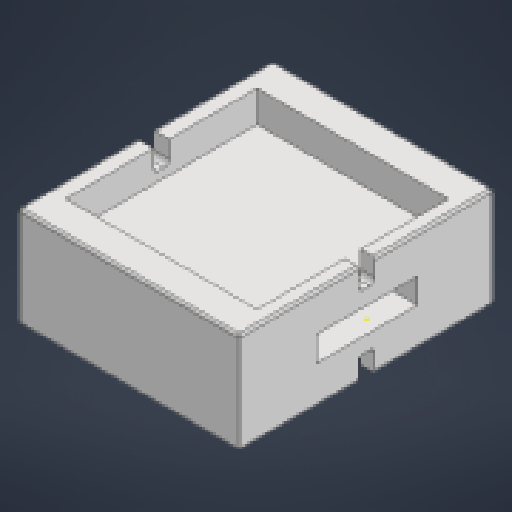
# Autodesk Inventor part: Base_Casing_A0645_v2
Saved by Autodesk Inventor 2026.2 (Build 302298000, 298)
## iProperties
Created: 2025-09-05
Part Number: Base_Casing_A0645_v2
Material: Generic
Document SubType Name: Modeling
Designer: usman
Density: 1 g/cm^3
Appearance: Default
Author: usman
Autodesk Inventor part; units mm, degrees
ref_plane "YZ Plane" through (0, 0, 0) normal (1, 0, 0) x (0, 1, 0)
ref_plane "XZ Plane" through (0, 0, 0) normal (0, 1, 0) x (-1, 0, 0)
ref_plane "XY Plane" through (0, 0, 0) normal (0, 0, 1) x (1, 0, 0)
sketch "Sketch1" plane through (0, 0, 0) normal (1, 0, 0) x (0, 1, 0)
  line L0 (-20, 51) -> (20, 51)
  line L1 (20, 51) -> (20, -51)
  line L2 (20, -51) -> (-20, -51)
  line L3 (-20, -51) -> (-20, 51)
  line L4 (-20, 51) -> (20, -51) construction
  line L5 (20, 51) -> (-20, -51) construction
  point P0 (0, 0)
  dimension "d0" = 40
  dimension "d30" = 102
  constraints: 12 end point, 2 midpoint, 2 parallel, 1 horizontal, 1 perpendicular
  measures "d0" distance of L1.end L2.end
  measures "d30" distance of L2.end L0.start
extrude "Extrusion1" add sketch "Sketch1" along normal blind 88.5
sketch "Sketch2" plane through (88.5, 0, 0) normal (1, 0, 0) x (0, 0, -1)
  line L0 (-20.32, -5) -> (20.32, -5)
  line L1 (20.32, -5) -> (20.32, 5)
  line L2 (20.32, 5) -> (-20.32, 5)
  line L3 (-20.32, 5) -> (-20.32, -5)
  line L4 (-20.32, -5) -> (20.32, 5) construction
  line L5 (20.32, -5) -> (-20.32, 5) construction
  point P0 (0, 0)
  dimension "d4" = 10
  dimension "d5" = 40.64
  constraints: 12 end point, 2 midpoint, 2 parallel, 1 horizontal, 1 perpendicular
  measures "d4" distance of L0.end L1.end
  measures "d5" distance of L1.end L2.end
extrude "Extrusion2" cut sketch "Sketch2" against normal through all
sketch "Sketch3" plane through (88.5, 0, 0) normal (1, 0, 0) x (0, 0, -1)
  point P0 (0, 0)
sketch "Sketch4" plane through (0, 20, 51) normal (0, 1, 0) x (1, 0, 0)
  line L0 (0, 102) -> (0, 0) projected
  line L1 (0, 102) -> (88.5, 102) projected
  line L2 (6.4418, 89.25) -> (82.9418, 89.25)
  line L3 (82.9418, 89.25) -> (82.9418, 12.75)
  line L4 (82.9418, 12.75) -> (6.4418, 12.75)
  line L5 (6.4418, 12.75) -> (6.4418, 89.25)
  line L6 (6.4418, 89.25) -> (82.9418, 12.75) construction
  line L7 (82.9418, 89.25) -> (6.4418, 12.75) construction
  line L8 (0, 0) -> (88.5, 0) projected
  point P0 (0, 51)
  point P1 (44.6918, 51)
  dimension "d24" = 102
  dimension "d31" = 76.5
  dimension "d32" = 76.5
  dimension "d34" = 51
  constraints: 12 end point, 2 parallel, 1 horizontal, 1 midpoint, 1 perpendicular
  measures "d24" distance of L0.start L0.end
  measures "d31" distance of L3.end L4.end
  measures "d32" distance of L2.end L3.end
  measures "d34" distance from line of L8 point (44.692, 51)
extrude "Extrusion3" cut sketch "Sketch4" against normal blind 12.5
mirror "Mirror1" about plane through (0, 0, 0) normal (0, 1, 0) of "Extrusion3"
sketch "Sketch5" plane through (0, 0, 0) normal (-1, 0, 0) x (0, 0, 1)
  line L0 (-51, 20) -> (51, 20) projected
  line L1 (-3.25, 11) -> (3.25, 11)
  line L2 (3.25, 11) -> (3.25, 20)
  line L3 (3.25, 20) -> (-3.25, 20)
  line L4 (-3.25, 20) -> (-3.25, 11)
  line L5 (-3.25, 11) -> (3.25, 20) construction
  line L6 (3.25, 11) -> (-3.25, 20) construction
  point P0 (0, 0)
  point P1 (0, 15.5)
  point P2 (-3.25, 20)
  dimension "d12" = 3.25
  dimension "d13" = 9
  constraints: 12 end point, 2 midpoint, 2 parallel, 1 horizontal, 1 perpendicular, 1 point on line
  measures "d12" distance from line of point (0, 15.5) L2
  measures "d13" distance of L1.end L2.end
extrude "Extrusion4" cut sketch "Sketch5" against normal through all
mirror "Mirror2" about plane through (0, 0, 0) normal (0, 1, 0) of "Extrusion4"
sketch "Sketch6" plane through (0, 0, 0) normal (-1, 0, 0) x (0, 0, 1)
  line L0 (-39.5306, -14.8221) -> (-39.5306, 14.9585) construction
  line L1 (-39.5306, 14.9585) -> (-30.121, 14.9585) construction
  line L2 (-30.121, 14.9585) -> (-30.121, -14.8221) construction
  line L3 (-30.121, -14.8221) -> (-39.5306, -14.8221) construction
  line L4 (-39.3809, -5.65) -> (-43.1909, -5.65)
  line L5 (-43.1909, -5.65) -> (-43.1909, -5.0532)
  spline S0 degree 2 poles (-43.1909, -5.0532) (-43.1909, -4.5318) (-43.125, -4.2899) knots 0 0 0 1 1 1
  spline S1 degree 2 poles (-43.125, -4.2899) (-43.0339, -3.9507) (-42.5407, -3.5455) (-42.2078, -3.5455) knots 0 0 0 1 2 2 2
  spline S2 degree 2 poles (-42.2078, -3.5455) (-41.9879, -3.5455) (-41.633, -3.7277) (-41.4791, -3.935) knots 0 0 0 1 2 2 2
  spline S3 degree 2 poles (-41.4791, -3.935) (-41.3158, -3.5863) (-40.8258, -3.266) (-40.4928, -3.266) knots 0 0 0 1 2 2 2
  spline S4 degree 2 poles (-40.4928, -3.266) (-40.1693, -3.266) (-39.6416, -3.5989) (-39.3809, -4.1203) (-39.3809, -4.582) knots 0 0 0 1 2 3 3 3
  line L6 (-39.3809, -4.582) -> (-39.3809, -5.65)
  line L7 (-41.0488, -4.9244) -> (-40.0719, -4.9244)
  line L8 (-40.0719, -4.9244) -> (-40.0719, -4.7422)
  spline S5 degree 2 poles (-40.0719, -4.7422) (-40.0719, -4.2931) (-40.3012, -3.979) (-40.518, -3.979) knots 0 0 0 1 2 2 2
  spline S6 degree 2 poles (-40.518, -3.979) (-40.7629, -3.979) (-41.0488, -4.3465) (-41.0488, -4.7736) knots 0 0 0 1 2 2 2
  line L9 (-41.0488, -4.7736) -> (-41.0488, -4.9244)
  line L10 (-42.4999, -4.9244) -> (-41.6958, -4.9244)
  line L11 (-41.6958, -4.9244) -> (-41.6958, -4.7673)
  spline S7 degree 2 poles (-41.6958, -4.7673) (-41.6958, -4.5035) (-41.9188, -4.2459) (-42.1104, -4.2459) knots 0 0 0 1 2 2 2
  spline S8 degree 2 poles (-42.1104, -4.2459) (-42.2895, -4.2459) (-42.4999, -4.4878) (-42.4999, -4.7391) knots 0 0 0 1 2 2 2
  line L12 (-42.4999, -4.7391) -> (-42.4999, -4.9244)
  line L13 (-42.1984, -0.571) -> (-42.1984, 0.1357)
  line L14 (-42.1984, 0.1357) -> (-39.3809, 0.1357)
  line L15 (-39.3809, 0.1357) -> (-39.3809, -0.571)
  line L16 (-39.3809, -0.571) -> (-39.6793, -0.571)
  spline S9 degree 2 poles (-39.6793, -0.571) (-39.4814, -0.7783) (-39.3087, -1.1929) (-39.3087, -1.4379) knots 0 0 0 1 2 2 2
  spline S10 degree 2 poles (-39.3087, -1.4379) (-39.3087, -1.9813) (-40.1567, -2.7791) (-40.7849, -2.7791) knots 0 0 0 1 2 2 2
  spline S11 degree 2 poles (-40.7849, -2.7791) (-41.4383, -2.7791) (-42.2706, -2.0096) (-42.2706, -1.4568) knots 0 0 0 1 2 2 2
  spline S12 degree 2 poles (-42.2706, -1.4568) (-42.2706, -1.2055) (-42.079, -0.7595) (-41.8874, -0.571) knots 0 0 0 1 2 2 2
  line L17 (-41.8874, -0.571) -> (-42.1984, -0.571)
  spline S13 degree 2 poles (-41.6173, -1.3154) (-41.6173, -1.6421) (-41.1556, -2.0755) (-40.7912, -2.0755) knots 0 0 0 1 2 2 2
  spline S14 degree 2 poles (-40.7912, -2.0755) (-40.4269, -2.0755) (-39.9557, -1.6327) (-39.9557, -1.3123) knots 0 0 0 1 2 2 2
  spline S15 degree 2 poles (-39.9557, -1.3123) (-39.9557, -0.9793) (-40.4206, -0.5396) (-40.7944, -0.5396) knots 0 0 0 1 2 2 2
  spline S16 degree 2 poles (-40.7944, -0.5396) (-41.1619, -0.5396) (-41.6173, -0.9793) (-41.6173, -1.3154) knots 0 0 0 1 2 2 2
  line L18 (-41.8026, 2.5731) -> (-41.366, 2.1365)
  spline S17 degree 2 poles (-41.366, 2.1365) (-41.6299, 1.8727) (-41.6299, 1.6559) knots 0 0 0 1 1 1
  spline S18 degree 2 poles (-41.6299, 1.6559) (-41.6299, 1.5366) (-41.5293, 1.4015) (-41.454, 1.4015) knots 0 0 0 1 2 2 2
  spline S19 degree 2 poles (-41.454, 1.4015) (-41.3974, 1.4015) (-41.3001, 1.4863) (-41.2184, 1.6559) knots 0 0 0 1 2 2 2
  line L19 (-41.2184, 1.6559) -> (-41.0896, 1.9135)
  spline S20 degree 2 poles (-41.0896, 1.9135) (-40.8886, 2.3218) (-40.4677, 2.6265) (-40.185, 2.6265) knots 0 0 0 1 2 2 2
  spline S21 degree 2 poles (-40.185, 2.6265) (-39.8112, 2.6265) (-39.3087, 2.0768) (-39.3087, 1.612) knots 0 0 0 1 2 2 2
  spline S22 degree 2 poles (-39.3087, 1.612) (-39.3087, 0.9963) (-39.7892, 0.6288) knots 0 0 0 1 1 1
  line L20 (-39.7892, 0.6288) -> (-40.2635, 1.0623)
  spline S23 degree 2 poles (-40.2635, 1.0623) (-40.119, 1.1879) (-39.94, 1.5209) (-39.94, 1.6497) knots 0 0 0 1 2 2 2
  spline S24 degree 2 poles (-39.94, 1.6497) (-39.94, 1.791) (-40.0751, 1.9606) (-40.163, 1.9606) knots 0 0 0 1 2 2 2
  spline S25 degree 2 poles (-40.163, 1.9606) (-40.3264, 1.9606) (-40.4803, 1.6528) knots 0 0 0 1 1 1
  line L21 (-40.4803, 1.6528) -> (-40.5996, 1.4141)
  spline S26 degree 2 poles (-40.5996, 1.4141) (-40.9451, 0.7325) (-41.4634, 0.7325) knots 0 0 0 1 1 1
  spline S27 degree 2 poles (-41.4634, 0.7325) (-41.7963, 0.7325) (-42.2706, 1.2476) (-42.2706, 1.6465) knots 0 0 0 1 2 2 2
  spline S28 degree 2 poles (-42.2706, 1.6465) (-42.2706, 1.9229) (-42.0288, 2.4066) (-41.8026, 2.5731) knots 0 0 0 1 2 2 2
  line L22 (-40.5871, 6.0062) -> (-40.5871, 3.7384)
  spline S29 degree 2 poles (-40.5871, 3.7384) (-40.2855, 3.7887) (-39.9306, 4.2158) (-39.9306, 4.5456) knots 0 0 0 1 2 2 2
  spline S30 degree 2 poles (-39.9306, 4.5456) (-39.9306, 4.9414) (-40.207, 5.2272) knots 0 0 0 1 1 1
  line L23 (-40.207, 5.2272) -> (-39.9274, 5.8209)
  spline S31 degree 2 poles (-39.9274, 5.8209) (-39.6134, 5.5979) (-39.3087, 4.976) (-39.3087, 4.5488) knots 0 0 0 1 2 2 2
  spline S32 degree 2 poles (-39.3087, 4.5488) (-39.3087, 3.886) (-40.1442, 3.0537) (-40.7755, 3.0537) knots 0 0 0 1 2 2 2
  spline S33 degree 2 poles (-40.7755, 3.0537) (-41.4194, 3.0537) (-42.2706, 3.886) (-42.2706, 4.5111) knots 0 0 0 1 2 2 2
  spline S34 degree 2 poles (-42.2706, 4.5111) (-42.2706, 5.177) (-41.4194, 6.0093) (-40.7221, 6.0093) knots 0 0 0 1 2 2 2
  line L24 (-40.7221, 6.0093) -> (-40.5871, 6.0062)
  spline S35 degree 2 poles (-41.143, 5.2995) (-41.3786, 5.2304) (-41.6707, 4.8189) (-41.6707, 4.5456) knots 0 0 0 1 2 2 2
  spline S36 degree 2 poles (-41.6707, 4.5456) (-41.6707, 4.2504) (-41.5074, 4.0274) knots 0 0 0 1 1 1
  spline S37 degree 2 poles (-41.5074, 4.0274) (-41.4037, 3.8892) (-41.143, 3.7698) knots 0 0 0 1 1 1
  line L25 (-41.143, 3.7698) -> (-41.143, 5.2995)
  line L26 (-36.7148, -15.7859) -> (-36.7148, -15.0823)
  line L27 (-36.7148, -15.0823) -> (-34.0575, -14.1965)
  line L28 (-34.0575, -14.1965) -> (-36.7148, -13.3045)
  line L29 (-36.7148, -13.3045) -> (-36.7148, -12.6009)
  line L30 (-36.7148, -12.6009) -> (-32.9048, -11.9633)
  line L31 (-32.9048, -11.9633) -> (-32.9048, -12.6638)
  line L32 (-32.9048, -12.6638) -> (-35.3108, -13.0689)
  line L33 (-35.3108, -13.0689) -> (-32.9048, -13.8793)
  line L34 (-32.9048, -13.8793) -> (-32.9048, -14.5201)
  line L35 (-32.9048, -14.5201) -> (-35.3108, -15.321)
  line L36 (-35.3108, -15.321) -> (-32.9048, -15.7388)
  line L37 (-32.9048, -15.7388) -> (-32.9048, -16.4455)
  line L38 (-32.9048, -16.4455) -> (-36.7148, -15.7859)
  line L39 (-35.7222, -9.3783) -> (-35.7222, -8.6716)
  line L40 (-35.7222, -8.6716) -> (-32.9048, -8.6716)
  line L41 (-32.9048, -8.6716) -> (-32.9048, -9.3783)
  line L42 (-32.9048, -9.3783) -> (-33.2032, -9.3783)
  spline S38 degree 2 poles (-33.2032, -9.3783) (-33.0053, -9.5856) (-32.8325, -10.0002) (-32.8325, -10.2452) knots 0 0 0 1 2 2 2
  spline S39 degree 2 poles (-32.8325, -10.2452) (-32.8325, -10.7886) (-33.6806, -11.5864) (-34.3088, -11.5864) knots 0 0 0 1 2 2 2
  spline S40 degree 2 poles (-34.3088, -11.5864) (-34.9621, -11.5864) (-35.7945, -10.8169) (-35.7945, -10.2641) knots 0 0 0 1 2 2 2
  spline S41 degree 2 poles (-35.7945, -10.2641) (-35.7945, -10.0128) (-35.6029, -9.5668) (-35.4113, -9.3783) knots 0 0 0 1 2 2 2
  line L43 (-35.4113, -9.3783) -> (-35.7222, -9.3783)
  spline S42 degree 2 poles (-35.1412, -10.1227) (-35.1412, -10.4494) (-34.6794, -10.8828) (-34.3151, -10.8828) knots 0 0 0 1 2 2 2
  spline S43 degree 2 poles (-34.3151, -10.8828) (-33.9507, -10.8828) (-33.4796, -10.4399) (-33.4796, -10.1196) knots 0 0 0 1 2 2 2
  spline S44 degree 2 poles (-33.4796, -10.1196) (-33.4796, -9.7866) (-33.9445, -9.3469) (-34.3182, -9.3469) knots 0 0 0 1 2 2 2
  spline S45 degree 2 poles (-34.3182, -9.3469) (-34.6857, -9.3469) (-35.1412, -9.7866) (-35.1412, -10.1227) knots 0 0 0 1 2 2 2
  line L44 (-35.7222, -5.8761) -> (-35.7222, -5.1694)
  line L45 (-35.7222, -5.1694) -> (-33.31, -5.1694)
  spline S46 degree 2 poles (-33.31, -5.1694) (-32.5938, -5.1694) (-32.2577, -5.4584) knots 0 0 0 1 1 1
  spline S47 degree 2 poles (-32.2577, -5.4584) (-31.8023, -5.8416) (-31.8023, -6.6205) knots 0 0 0 1 1 1
  spline S48 degree 2 poles (-31.8023, -6.6205) (-31.8023, -7.0351) (-32.0096, -7.5974) (-32.4117, -7.9868) (-32.6975, -8.0811) knots 0 0 0 1 2 3 3 3
  line L46 (-32.6975, -8.0811) -> (-32.6975, -7.3021)
  spline S49 degree 2 poles (-32.6975, -7.3021) (-32.5781, -7.1985) (-32.4588, -6.8718) (-32.4588, -6.6488) knots 0 0 0 1 2 2 2
  spline S50 degree 2 poles (-32.4588, -6.6488) (-32.4588, -6.3661) (-32.6347, -6.0175) (-32.9142, -5.8761) (-33.2566, -5.8761) knots 0 0 0 1 2 3 3 3
  spline S51 degree 2 poles (-33.2566, -5.8761) (-33.0681, -6.0614) (-32.9048, -6.4698) (-32.9048, -6.7305) knots 0 0 0 1 2 2 2
  spline S52 degree 2 poles (-32.9048, -6.7305) (-32.9048, -7.2958) (-33.7246, -8.0779) (-34.3496, -8.0779) knots 0 0 0 1 2 2 2
  spline S53 degree 2 poles (-34.3496, -8.0779) (-35.0218, -8.0779) (-35.427, -7.6633) knots 0 0 0 1 1 1
  spline S54 degree 2 poles (-35.427, -7.6633) (-35.7945, -7.2895) (-35.7945, -6.7681) knots 0 0 0 1 1 1
  spline S55 degree 2 poles (-35.7945, -6.7681) (-35.7945, -6.5263) (-35.6154, -6.0928) (-35.4113, -5.8761) knots 0 0 0 1 2 2 2
  line L47 (-35.4113, -5.8761) -> (-35.7222, -5.8761)
  spline S56 degree 2 poles (-35.1349, -6.6048) (-35.1349, -6.9409) (-34.6857, -7.3744) (-34.3465, -7.3744) knots 0 0 0 1 2 2 2
  spline S57 degree 2 poles (-34.3465, -7.3744) (-33.9947, -7.3744) (-33.5455, -6.9283) (-33.5455, -6.5923) knots 0 0 0 1 2 2 2
  spline S58 degree 2 poles (-33.5455, -6.5923) (-33.5455, -6.2656) (-33.9853, -5.8384) (-34.3434, -5.8384) knots 0 0 0 1 2 2 2
  spline S59 degree 2 poles (-34.3434, -5.8384) (-34.6951, -5.8384) (-35.1349, -6.2687) (-35.1349, -6.6048) knots 0 0 0 1 2 2 2
  line L48 (-35.7222, -4.4533) -> (-35.7222, -3.7465)
  line L49 (-35.7222, -3.7465) -> (-35.4333, -3.7465)
  spline S60 degree 2 poles (-35.4333, -3.7465) (-35.6374, -3.5047) (-35.7945, -3.1152) (-35.7945, -2.911) knots 0 0 0 1 2 2 2
  spline S61 degree 2 poles (-35.7945, -2.911) (-35.7945, -2.4901) (-35.5024, -2.198) knots 0 0 0 1 1 1
  spline S62 degree 2 poles (-35.5024, -2.198) (-35.2542, -1.953) (-34.7674, -1.953) knots 0 0 0 1 1 1
  line L50 (-34.7674, -1.953) -> (-32.9048, -1.953)
  line L51 (-32.9048, -1.953) -> (-32.9048, -2.6535)
  line L52 (-32.9048, -2.6535) -> (-34.1392, -2.6535)
  spline S63 degree 2 poles (-34.1392, -2.6535) (-34.6417, -2.6535) (-34.9747, -2.7446) (-35.1474, -2.9676) (-35.1474, -3.134) knots 0 0 0 1 2 3 3 3
  spline S64 degree 2 poles (-35.1474, -3.134) (-35.1474, -3.3476) (-34.8616, -3.6554) (-34.6072, -3.7151) knots 0 0 0 1 2 2 2
  spline S65 degree 2 poles (-34.6072, -3.7151) (-34.4753, -3.7465) (-34.0355, -3.7465) knots 0 0 0 1 1 1
  line L53 (-34.0355, -3.7465) -> (-32.9048, -3.7465)
  line L54 (-32.9048, -3.7465) -> (-32.9048, -4.4533)
  line L55 (-32.9048, -4.4533) -> (-35.7222, -4.4533)
  line L56 (-34.1109, 1.5523) -> (-34.1109, -0.7155)
  spline S66 degree 2 poles (-34.1109, -0.7155) (-33.8094, -0.6652) (-33.4545, -0.2381) (-33.4545, 0.0917) knots 0 0 0 1 2 2 2
  spline S67 degree 2 poles (-33.4545, 0.0917) (-33.4545, 0.4875) (-33.7309, 0.7733) knots 0 0 0 1 1 1
  line L57 (-33.7309, 0.7733) -> (-33.4513, 1.367)
  spline S68 degree 2 poles (-33.4513, 1.367) (-33.1372, 1.144) (-32.8325, 0.5221) (-32.8325, 0.0949) knots 0 0 0 1 2 2 2
  spline S69 degree 2 poles (-32.8325, 0.0949) (-32.8325, -0.5679) (-33.668, -1.4002) (-34.2994, -1.4002) knots 0 0 0 1 2 2 2
  spline S70 degree 2 poles (-34.2994, -1.4002) (-34.9433, -1.4002) (-35.7945, -0.5679) (-35.7945, 0.0572) knots 0 0 0 1 2 2 2
  spline S71 degree 2 poles (-35.7945, 0.0572) (-35.7945, 0.7231) (-34.9433, 1.5554) (-34.246, 1.5554) knots 0 0 0 1 2 2 2
  line L58 (-34.246, 1.5554) -> (-34.1109, 1.5523)
  spline S72 degree 2 poles (-34.6669, 0.8456) (-34.9024, 0.7765) (-35.1946, 0.365) (-35.1946, 0.0917) knots 0 0 0 1 2 2 2
  spline S73 degree 2 poles (-35.1946, 0.0917) (-35.1946, -0.2035) (-35.0312, -0.4265) knots 0 0 0 1 1 1
  spline S74 degree 2 poles (-35.0312, -0.4265) (-34.9276, -0.5647) (-34.6669, -0.6841) knots 0 0 0 1 1 1
  line L59 (-34.6669, -0.6841) -> (-34.6669, 0.8456)
  line L60 (-36.7619, 2.2119) -> (-36.7619, 2.9186)
  line L61 (-36.7619, 2.9186) -> (-35.7222, 2.9186)
  line L62 (-35.7222, 2.9186) -> (-35.7222, 3.3395)
  line L63 (-35.7222, 3.3395) -> (-35.1129, 3.3395)
  line L64 (-35.1129, 3.3395) -> (-35.1129, 2.9186)
  line L65 (-35.1129, 2.9186) -> (-32.9048, 2.9186)
  line L66 (-32.9048, 2.9186) -> (-32.9048, 2.2119)
  line L67 (-32.9048, 2.2119) -> (-35.1129, 2.2119)
  line L68 (-35.1129, 2.2119) -> (-35.1129, 1.8507)
  line L69 (-35.1129, 1.8507) -> (-35.7222, 1.8507)
  line L70 (-35.7222, 1.8507) -> (-35.7222, 2.2119)
  line L71 (-35.7222, 2.2119) -> (-36.7619, 2.2119)
  line L72 (-36.0426, 7.294) -> (-35.5589, 6.7883)
  spline S75 degree 2 poles (-35.5589, 6.7883) (-36.1054, 6.27) (-36.1054, 5.623) knots 0 0 0 1 1 1
  spline S76 degree 2 poles (-36.1054, 5.623) (-36.1054, 5.0765) (-35.361, 4.3289) (-34.8145, 4.3289) knots 0 0 0 1 2 2 2
  spline S77 degree 2 poles (-34.8145, 4.3289) (-34.4344, 4.3289) (-33.8439, 4.6587) (-33.5079, 5.2649) (-33.5079, 5.6356) knots 0 0 0 1 2 3 3 3
  spline S78 degree 2 poles (-33.5079, 5.6356) (-33.5079, 5.9497) (-33.7434, 6.4742) (-34.0544, 6.7883) knots 0 0 0 1 2 2 2
  line L73 (-34.0544, 6.7883) -> (-33.5424, 7.2783)
  spline S79 degree 2 poles (-33.5424, 7.2783) (-33.1278, 6.8574) (-32.8106, 6.1067) (-32.8106, 5.623) knots 0 0 0 1 2 2 2
  spline S80 degree 2 poles (-32.8106, 5.623) (-32.8106, 4.7341) (-33.935, 3.6033) (-34.8176, 3.6033) knots 0 0 0 1 2 2 2
  spline S81 degree 2 poles (-34.8176, 3.6033) (-35.3862, 3.6033) (-36.2719, 4.1185) (-36.809, 5.0796) (-36.809, 5.6324) knots 0 0 0 1 2 3 3 3
  spline S82 degree 2 poles (-36.809, 5.6324) (-36.809, 6.1067) (-36.4101, 6.9768) (-36.0426, 7.294) knots 0 0 0 1 2 2 2
  line L74 (-35.7222, 9.9324) -> (-35.7222, 10.6391)
  line L75 (-35.7222, 10.6391) -> (-32.9048, 10.6391)
  line L76 (-32.9048, 10.6391) -> (-32.9048, 9.9324)
  line L77 (-32.9048, 9.9324) -> (-33.2032, 9.9324)
  spline S83 degree 2 poles (-33.2032, 9.9324) (-33.0053, 9.7251) (-32.8325, 9.3105) (-32.8325, 9.0655) knots 0 0 0 1 2 2 2
  spline S84 degree 2 poles (-32.8325, 9.0655) (-32.8325, 8.5221) (-33.6806, 7.7243) (-34.3088, 7.7243) knots 0 0 0 1 2 2 2
  spline S85 degree 2 poles (-34.3088, 7.7243) (-34.9621, 7.7243) (-35.7945, 8.4938) (-35.7945, 9.0467) knots 0 0 0 1 2 2 2
  spline S86 degree 2 poles (-35.7945, 9.0467) (-35.7945, 9.2979) (-35.6029, 9.7439) (-35.4113, 9.9324) knots 0 0 0 1 2 2 2
  line L78 (-35.4113, 9.9324) -> (-35.7222, 9.9324)
  spline S87 degree 2 poles (-35.1412, 9.188) (-35.1412, 8.8613) (-34.6794, 8.4279) (-34.3151, 8.4279) knots 0 0 0 1 2 2 2
  spline S88 degree 2 poles (-34.3151, 8.4279) (-33.9507, 8.4279) (-33.4796, 8.8708) (-33.4796, 9.1911) knots 0 0 0 1 2 2 2
  spline S89 degree 2 poles (-33.4796, 9.1911) (-33.4796, 9.5241) (-33.9445, 9.9638) (-34.3182, 9.9638) knots 0 0 0 1 2 2 2
  spline S90 degree 2 poles (-34.3182, 9.9638) (-34.6857, 9.9638) (-35.1412, 9.5241) (-35.1412, 9.188) knots 0 0 0 1 2 2 2
  line L79 (-35.3265, 13.0765) -> (-34.8899, 12.6399)
  spline S91 degree 2 poles (-34.8899, 12.6399) (-35.1537, 12.3761) (-35.1537, 12.1594) knots 0 0 0 1 1 1
  spline S92 degree 2 poles (-35.1537, 12.1594) (-35.1537, 12.04) (-35.0532, 11.9049) (-34.9778, 11.9049) knots 0 0 0 1 2 2 2
  spline S93 degree 2 poles (-34.9778, 11.9049) (-34.9213, 11.9049) (-34.8239, 11.9897) (-34.7423, 12.1594) knots 0 0 0 1 2 2 2
  line L80 (-34.7423, 12.1594) -> (-34.6135, 12.4169)
  spline S94 degree 2 poles (-34.6135, 12.4169) (-34.4125, 12.8252) (-33.9916, 13.1299) (-33.7089, 13.1299) knots 0 0 0 1 2 2 2
  spline S95 degree 2 poles (-33.7089, 13.1299) (-33.3351, 13.1299) (-32.8325, 12.5802) (-32.8325, 12.1154) knots 0 0 0 1 2 2 2
  spline S96 degree 2 poles (-32.8325, 12.1154) (-32.8325, 11.4998) (-33.3131, 11.1323) knots 0 0 0 1 1 1
  line L81 (-33.3131, 11.1323) -> (-33.7874, 11.5657)
  spline S97 degree 2 poles (-33.7874, 11.5657) (-33.6429, 11.6914) (-33.4639, 12.0243) (-33.4639, 12.1531) knots 0 0 0 1 2 2 2
  spline S98 degree 2 poles (-33.4639, 12.1531) (-33.4639, 12.2944) (-33.5989, 12.464) (-33.6869, 12.464) knots 0 0 0 1 2 2 2
  spline S99 degree 2 poles (-33.6869, 12.464) (-33.8502, 12.464) (-34.0041, 12.1562) knots 0 0 0 1 1 1
  line L82 (-34.0041, 12.1562) -> (-34.1235, 11.9175)
  spline S100 degree 2 poles (-34.1235, 11.9175) (-34.469, 11.2359) (-34.9873, 11.2359) knots 0 0 0 1 1 1
  spline S101 degree 2 poles (-34.9873, 11.2359) (-35.3202, 11.2359) (-35.7945, 11.751) (-35.7945, 12.1499) knots 0 0 0 1 2 2 2
  spline S102 degree 2 poles (-35.7945, 12.1499) (-35.7945, 12.4263) (-35.5526, 12.91) (-35.3265, 13.0765) knots 0 0 0 1 2 2 2
  line L83 (-34.1109, 16.5096) -> (-34.1109, 14.2418)
  spline S103 degree 2 poles (-34.1109, 14.2418) (-33.8094, 14.2921) (-33.4545, 14.7192) (-33.4545, 15.0491) knots 0 0 0 1 2 2 2
  spline S104 degree 2 poles (-33.4545, 15.0491) (-33.4545, 15.4448) (-33.7309, 15.7306) knots 0 0 0 1 1 1
  line L84 (-33.7309, 15.7306) -> (-33.4513, 16.3243)
  spline S105 degree 2 poles (-33.4513, 16.3243) (-33.1372, 16.1013) (-32.8325, 15.4794) (-32.8325, 15.0522) knots 0 0 0 1 2 2 2
  spline S106 degree 2 poles (-32.8325, 15.0522) (-32.8325, 14.3894) (-33.668, 13.5571) (-34.2994, 13.5571) knots 0 0 0 1 2 2 2
  spline S107 degree 2 poles (-34.2994, 13.5571) (-34.9433, 13.5571) (-35.7945, 14.3894) (-35.7945, 15.0145) knots 0 0 0 1 2 2 2
  spline S108 degree 2 poles (-35.7945, 15.0145) (-35.7945, 15.6804) (-34.9433, 16.5127) (-34.246, 16.5127) knots 0 0 0 1 2 2 2
  line L85 (-34.246, 16.5127) -> (-34.1109, 16.5096)
  spline S109 degree 2 poles (-34.6669, 15.8029) (-34.9024, 15.7338) (-35.1946, 15.3223) (-35.1946, 15.0491) knots 0 0 0 1 2 2 2
  spline S110 degree 2 poles (-35.1946, 15.0491) (-35.1946, 14.7538) (-35.0312, 14.5308) knots 0 0 0 1 1 1
  spline S111 degree 2 poles (-35.0312, 14.5308) (-34.9276, 14.3926) (-34.6669, 14.2732) knots 0 0 0 1 1 1
  line L86 (-34.6669, 14.2732) -> (-34.6669, 15.8029)
  line L87 (-26.541, -8.4163) -> (-30.351, -7.1288)
  line L88 (-30.351, -7.1288) -> (-30.351, -6.0852)
  line L89 (-30.351, -6.0852) -> (-26.541, -4.7978)
  line L90 (-26.541, -4.7978) -> (-26.541, -5.7827)
  line L91 (-26.541, -5.7827) -> (-27.319, -6.0204)
  line L92 (-27.319, -6.0204) -> (-27.319, -7.2184)
  line L93 (-27.319, -7.2184) -> (-26.541, -7.4592)
  line L94 (-26.541, -7.4592) -> (-26.541, -8.4163)
  line L95 (-28.0106, -6.2304) -> (-29.2703, -6.6194)
  line L96 (-29.2703, -6.6194) -> (-28.0106, -7.0115)
  line L97 (-28.0106, -7.0115) -> (-28.0106, -6.2304)
  spline S112 degree 2 poles (-28.446, -1.6763) (-27.9519, -1.6763) (-27.2109, -1.8337) (-26.9609, -2.0097) knots 0 0 0 1 2 2 2
  spline S113 degree 2 poles (-26.9609, -2.0097) (-26.7139, -2.1826) (-26.4607, -2.7415) (-26.4607, -3.1428) knots 0 0 0 1 2 2 2
  spline S114 degree 2 poles (-26.4607, -3.1428) (-26.4607, -3.5473) (-26.7139, -4.1031) (-26.967, -4.279) knots 0 0 0 1 2 2 2
  spline S115 degree 2 poles (-26.967, -4.279) (-27.2171, -4.455) (-27.9519, -4.6125) (-28.446, -4.6125) knots 0 0 0 1 2 2 2
  spline S116 degree 2 poles (-28.446, -4.6125) (-28.9523, -4.6125) (-29.6686, -4.455) (-29.928, -4.276) knots 0 0 0 1 2 2 2
  spline S117 degree 2 poles (-29.928, -4.276) (-30.1811, -4.0969) (-30.4281, -3.5319) (-30.4281, -3.1428) knots 0 0 0 1 2 2 2
  spline S118 degree 2 poles (-30.4281, -3.1428) (-30.4281, -2.7322) (-30.1688, -2.1826) (-29.9125, -2.0066) knots 0 0 0 1 2 2 2
  spline S119 degree 2 poles (-29.9125, -2.0066) (-29.6624, -1.8337) (-28.9245, -1.6763) (-28.446, -1.6763) knots 0 0 0 1 2 2 2
  spline S120 degree 2 poles (-28.446, -2.6365) (-29.153, -2.6365) (-29.7242, -2.8681) (-29.7242, -3.1428) knots 0 0 0 1 2 2 2
  spline S121 degree 2 poles (-29.7242, -3.1428) (-29.7242, -3.4176) (-29.153, -3.6523) (-28.4429, -3.6523) knots 0 0 0 1 2 2 2
  spline S122 degree 2 poles (-28.4429, -3.6523) (-27.7451, -3.6523) (-27.1646, -3.4176) (-27.1646, -3.1428) knots 0 0 0 1 2 2 2
  spline S123 degree 2 poles (-27.1646, -3.1428) (-27.1646, -2.8711) (-27.7451, -2.6365) (-28.446, -2.6365) knots 0 0 0 1 2 2 2
  spline S124 degree 2 poles (-27.6957, 1.615) (-27.4147, 1.615) (-26.9547, 1.4082) (-26.7941, 1.2075) knots 0 0 0 1 2 2 2
  spline S125 degree 2 poles (-26.7941, 1.2075) (-26.6336, 1.0068) (-26.4607, 0.4603) (-26.4607, 0.0682) knots 0 0 0 1 2 2 2
  spline S126 degree 2 poles (-26.4607, 0.0682) (-26.4607, -0.3764) (-26.6089, -1.0125) (-26.7015, -1.2131) knots 0 0 0 1 2 2 2
  line L98 (-26.7015, -1.2131) -> (-27.529, -1.2131)
  line L99 (-27.529, -1.2131) -> (-27.529, -1.1205)
  spline S127 degree 2 poles (-27.529, -1.1205) (-27.3962, -0.9106) (-27.1986, -0.3455) (-27.1986, -0.1109) knots 0 0 0 1 2 2 2
  spline S128 degree 2 poles (-27.1986, -0.1109) (-27.1986, 0.028) (-27.248, 0.3522) (-27.3283, 0.4634) knots 0 0 0 1 2 2 2
  spline S129 degree 2 poles (-27.3283, 0.4634) (-27.3931, 0.5498) (-27.5814, 0.6548) (-27.7513, 0.6548) knots 0 0 0 1 2 2 2
  spline S130 degree 2 poles (-27.7513, 0.6548) (-27.9211, 0.6548) (-28.1032, 0.5066) (-28.1465, 0.3831) knots 0 0 0 1 2 2 2
  spline S131 degree 2 poles (-28.1465, 0.3831) (-28.1897, 0.2596) (-28.199, -0.0831) (-28.199, -0.2159) knots 0 0 0 1 2 2 2
  line L100 (-28.199, -0.2159) -> (-28.199, -0.3795)
  line L101 (-28.199, -0.3795) -> (-28.8689, -0.3795)
  line L102 (-28.8689, -0.3795) -> (-28.8689, -0.2282)
  spline S132 degree 2 poles (-28.8689, -0.2282) (-28.8689, -0.0553) (-28.8998, 0.238) (-28.9461, 0.3399) knots 0 0 0 1 2 2 2
  spline S133 degree 2 poles (-28.9461, 0.3399) (-28.9955, 0.4418) (-29.1684, 0.556) (-29.3166, 0.556) knots 0 0 0 1 2 2 2
  spline S134 degree 2 poles (-29.3166, 0.556) (-29.434, 0.556) (-29.5791, 0.4479) (-29.6192, 0.3708) knots 0 0 0 1 2 2 2
  spline S135 degree 2 poles (-29.6192, 0.3708) (-29.6655, 0.2781) (-29.6964, 0.0311) (-29.6964, -0.0553) knots 0 0 0 1 2 2 2
  spline S136 degree 2 poles (-29.6964, -0.0553) (-29.6964, -0.1943) (-29.6316, -0.4876) (-29.5791, -0.6234) knots 0 0 0 1 2 2 2
  spline S137 degree 2 poles (-29.5791, -0.6234) (-29.5389, -0.7315) (-29.4093, -0.9661) (-29.3753, -1.0217) knots 0 0 0 1 2 2 2
  line L103 (-29.3753, -1.0217) -> (-29.3753, -1.102)
  line L104 (-29.3753, -1.102) -> (-30.1904, -1.102)
  spline S138 degree 2 poles (-30.1904, -1.102) (-30.2738, -0.9044) (-30.4312, -0.2375) (-30.4312, 0.1114) knots 0 0 0 1 2 2 2
  spline S139 degree 2 poles (-30.4312, 0.1114) (-30.4312, 0.451) (-30.3139, 0.9512) (-30.1997, 1.1272) knots 0 0 0 1 2 2 2
  spline S140 degree 2 poles (-30.1997, 1.1272) (-30.0793, 1.3217) (-29.7087, 1.5162) (-29.4772, 1.5162) knots 0 0 0 1 2 2 2
  spline S141 degree 2 poles (-29.4772, 1.5162) (-29.1499, 1.5162) (-28.6621, 1.1395) (-28.5911, 0.8308) knots 0 0 0 1 2 2 2
  line L105 (-28.5911, 0.8308) -> (-28.554, 0.8308)
  spline S142 degree 2 poles (-28.554, 0.8308) (-28.5355, 0.9666) (-28.4367, 1.226) (-28.3255, 1.3495) knots 0 0 0 1 2 2 2
  spline S143 degree 2 poles (-28.3255, 1.3495) (-28.2267, 1.4637) (-27.9118, 1.615) (-27.6957, 1.615) knots 0 0 0 1 2 2 2
  line L106 (-26.541, 5.0484) -> (-26.541, 2.248)
  line L107 (-26.541, 2.248) -> (-27.1615, 2.248)
  spline S144 degree 2 poles (-27.1615, 2.248) (-27.4456, 2.603) (-27.9458, 3.1711) (-28.1712, 3.3842) knots 0 0 0 1 2 2 2
  spline S145 degree 2 poles (-28.1712, 3.3842) (-28.4645, 3.6651) (-28.9122, 3.9152) (-29.1468, 3.9152) knots 0 0 0 1 2 2 2
  spline S146 degree 2 poles (-29.1468, 3.9152) (-29.4123, 3.9152) (-29.6964, 3.5972) (-29.6964, 3.3132) knots 0 0 0 1 2 2 2
  spline S147 degree 2 poles (-29.6964, 3.3132) (-29.6964, 3.1681) (-29.6254, 2.9087) (-29.5698, 2.7759) knots 0 0 0 1 2 2 2
  spline S148 degree 2 poles (-29.5698, 2.7759) (-29.5111, 2.6463) (-29.3876, 2.461) (-29.3568, 2.4147) knots 0 0 0 1 2 2 2
  line L108 (-29.3568, 2.4147) -> (-29.3568, 2.3406)
  line L109 (-29.3568, 2.3406) -> (-30.1873, 2.3406)
  spline S149 degree 2 poles (-30.1873, 2.3406) (-30.2645, 2.5011) (-30.4251, 3.1866) (-30.4251, 3.5046) knots 0 0 0 1 2 2 2
  spline S150 degree 2 poles (-30.4251, 3.5046) (-30.4251, 4.1838) (-29.8199, 4.8816) (-29.2734, 4.8816) knots 0 0 0 1 2 2 2
  spline S151 degree 2 poles (-29.2734, 4.8816) (-28.9369, 4.8816) (-28.2885, 4.5636) (-27.918, 4.1962) knots 0 0 0 1 2 2 2
  spline S152 degree 2 poles (-27.918, 4.1962) (-27.6895, 3.9646) (-27.3344, 3.5293) (-27.2603, 3.4336) knots 0 0 0 1 2 2 2
  line L110 (-27.2603, 3.4336) -> (-27.2603, 5.0484)
  line L111 (-27.2603, 5.0484) -> (-26.541, 5.0484)
  spline S153 degree 2 poles (-28.446, 8.3366) (-27.9519, 8.3366) (-27.2109, 8.1791) (-26.9609, 8.0031) knots 0 0 0 1 2 2 2
  spline S154 degree 2 poles (-26.9609, 8.0031) (-26.7139, 7.8302) (-26.4607, 7.2714) (-26.4607, 6.87) knots 0 0 0 1 2 2 2
  spline S155 degree 2 poles (-26.4607, 6.87) (-26.4607, 6.4655) (-26.7139, 5.9098) (-26.967, 5.7338) knots 0 0 0 1 2 2 2
  spline S156 degree 2 poles (-26.967, 5.7338) (-27.2171, 5.5578) (-27.9519, 5.4003) (-28.446, 5.4003) knots 0 0 0 1 2 2 2
  spline S157 degree 2 poles (-28.446, 5.4003) (-28.9523, 5.4003) (-29.6686, 5.5578) (-29.928, 5.7369) knots 0 0 0 1 2 2 2
  spline S158 degree 2 poles (-29.928, 5.7369) (-30.1811, 5.9159) (-30.4281, 6.481) (-30.4281, 6.87) knots 0 0 0 1 2 2 2
  spline S159 degree 2 poles (-30.4281, 6.87) (-30.4281, 7.2806) (-30.1688, 7.8302) (-29.9125, 8.0062) knots 0 0 0 1 2 2 2
  spline S160 degree 2 poles (-29.9125, 8.0062) (-29.6624, 8.1791) (-28.9245, 8.3366) (-28.446, 8.3366) knots 0 0 0 1 2 2 2
  spline S161 degree 2 poles (-28.446, 7.3763) (-29.153, 7.3763) (-29.7242, 7.1448) (-29.7242, 6.87) knots 0 0 0 1 2 2 2
  spline S162 degree 2 poles (-29.7242, 6.87) (-29.7242, 6.5952) (-29.153, 6.3605) (-28.4429, 6.3605) knots 0 0 0 1 2 2 2
  spline S163 degree 2 poles (-28.4429, 6.3605) (-27.7451, 6.3605) (-27.1646, 6.5952) (-27.1646, 6.87) knots 0 0 0 1 2 2 2
  spline S164 degree 2 poles (-27.1646, 6.87) (-27.1646, 7.1417) (-27.7451, 7.3763) (-28.446, 7.3763) knots 0 0 0 1 2 2 2
  point P0 (0, 0)
  dimension "d0" = 40
  dimension "d30" = 102
  constraints: 2 other
sketch "Sketch7" plane through (0, 0, 0) normal (-1, 0, 0) x (0, 0, 1)
  line L0 (10.5483, 19.7301) -> (34.9517, 19.7301) construction
  line L1 (34.9517, 19.7301) -> (34.9517, 12.5698) construction
  line L2 (34.9517, 12.5698) -> (10.5483, 12.5698) construction
  line L3 (10.5483, 12.5698) -> (10.5483, 19.7301) construction
  line L4 (-41.611, -7.2635) -> (-3.889, -7.2635) construction
  line L5 (-3.889, -7.2635) -> (-3.889, -18.9876) construction
  line L6 (-3.889, -18.9876) -> (-41.611, -18.9876) construction
  line L7 (-41.611, -18.9876) -> (-41.611, -7.2635) construction
  point P0 (0, 0)
  dimension "d0" = 40
  dimension "d30" = 102
  constraints: 4 other
sketch "Sketch8" plane through (0, 0, 0) normal (-1, 0, 0) x (0, 0, 1)
  line L0 (26.7591, -18.4593) -> (26.7591, 18.2389) construction
  line L1 (26.7591, 18.2389) -> (35.4697, 18.2389) construction
  line L2 (35.4697, 18.2389) -> (35.4697, -18.4593) construction
  line L3 (35.4697, -18.4593) -> (26.7591, -18.4593) construction
  spline S0 degree 2 poles (27.7193, -7.7114) (27.8826, -7.4538) (28.404, -7.1711) (28.7055, -7.1711) knots 0 0 0 1 2 2 2
  spline S1 degree 2 poles (28.7055, -7.1711) (29.0353, -7.1711) (29.5944, -7.5009) (29.8771, -8.0537) (29.8771, -8.4841) knots 0 0 0 1 2 3 3 3
  spline S2 degree 2 poles (29.8771, -8.4841) (29.8771, -8.9458) (29.6038, -9.4892) (29.0542, -9.8158) (28.7055, -9.8158) knots 0 0 0 1 2 3 3 3
  spline S3 degree 2 poles (28.7055, -9.8158) (28.4071, -9.8158) (27.9109, -9.5551) (27.7193, -9.2913) knots 0 0 0 1 2 2 2
  spline S4 degree 2 poles (27.7193, -9.2913) (27.5434, -9.464) (27.1539, -9.6368) (26.9372, -9.6368) knots 0 0 0 1 2 2 2
  spline S5 degree 2 poles (26.9372, -9.6368) (26.6388, -9.6368) (26.1488, -9.3478) (25.8786, -8.8296) (25.8786, -8.4903) knots 0 0 0 1 2 3 3 3
  spline S6 degree 2 poles (25.8786, -8.4903) (25.8786, -8.1574) (26.1519, -7.6486) (26.6576, -7.3565) (26.9466, -7.3565) knots 0 0 0 1 2 3 3 3
  spline S7 degree 2 poles (26.9466, -7.3565) (27.1507, -7.3565) (27.4994, -7.5104) (27.7193, -7.7114) knots 0 0 0 1 2 2 2
  spline S8 degree 2 poles (28.1056, -8.4872) (28.1056, -8.7479) (28.4228, -9.106) (28.6427, -9.106) knots 0 0 0 1 2 2 2
  spline S9 degree 2 poles (28.6427, -9.106) (28.872, -9.106) (29.1892, -8.7699) (29.1892, -8.4935) knots 0 0 0 1 2 2 2
  spline S10 degree 2 poles (29.1892, -8.4935) (29.1892, -8.2171) (28.894, -7.8873) (28.6584, -7.8873) knots 0 0 0 1 2 2 2
  spline S11 degree 2 poles (28.6584, -7.8873) (28.4228, -7.8873) (28.1056, -8.2296) (28.1056, -8.4872) knots 0 0 0 1 2 2 2
  spline S12 degree 2 poles (26.5791, -8.5155) (26.5791, -8.6945) (26.8147, -8.9238) (26.9968, -8.9238) knots 0 0 0 1 2 2 2
  spline S13 degree 2 poles (26.9968, -8.9238) (27.179, -8.9238) (27.4271, -8.6788) (27.4271, -8.5029) knots 0 0 0 1 2 2 2
  spline S14 degree 2 poles (27.4271, -8.5029) (27.4271, -8.3176) (27.1853, -8.082) (26.9905, -8.082) knots 0 0 0 1 2 2 2
  spline S15 degree 2 poles (26.9905, -8.082) (26.8084, -8.082) (26.5791, -8.3207) (26.5791, -8.5155) knots 0 0 0 1 2 2 2
  line L4 (25.9258, -6.5649) -> (25.9258, -5.8582)
  line L5 (25.9258, -5.8582) -> (26.9654, -5.8582)
  line L6 (26.9654, -5.8582) -> (26.9654, -5.4373)
  line L7 (26.9654, -5.4373) -> (27.5748, -5.4373)
  line L8 (27.5748, -5.4373) -> (27.5748, -5.8582)
  line L9 (27.5748, -5.8582) -> (29.7829, -5.8582)
  line L10 (29.7829, -5.8582) -> (29.7829, -6.5649)
  line L11 (29.7829, -6.5649) -> (27.5748, -6.5649)
  line L12 (27.5748, -6.5649) -> (27.5748, -6.9261)
  line L13 (27.5748, -6.9261) -> (26.9654, -6.9261)
  line L14 (26.9654, -6.9261) -> (26.9654, -6.5649)
  line L15 (26.9654, -6.5649) -> (25.9258, -6.5649)
  line L16 (25.8755, -5.0573) -> (25.8755, -4.3568)
  line L17 (25.8755, -4.3568) -> (27.2512, -4.3568)
  spline S16 degree 2 poles (27.2512, -4.3568) (27.0722, -4.1495) (26.8932, -3.7286) (26.8932, -3.515) knots 0 0 0 1 2 2 2
  spline S17 degree 2 poles (26.8932, -3.515) (26.8932, -3.0942) (27.1821, -2.8052) knots 0 0 0 1 1 1
  spline S18 degree 2 poles (27.1821, -2.8052) (27.4334, -2.5602) (27.9203, -2.5602) knots 0 0 0 1 1 1
  line L18 (27.9203, -2.5602) -> (29.7829, -2.5602)
  line L19 (29.7829, -2.5602) -> (29.7829, -3.2575)
  line L20 (29.7829, -3.2575) -> (28.5485, -3.2575)
  spline S19 degree 2 poles (28.5485, -3.2575) (28.0585, -3.2575) (27.7098, -3.3517) (27.5402, -3.5779) (27.5402, -3.7412) knots 0 0 0 1 2 3 3 3
  spline S20 degree 2 poles (27.5402, -3.7412) (27.5402, -3.9579) (27.826, -4.2657) (28.071, -4.3254) knots 0 0 0 1 2 2 2
  spline S21 degree 2 poles (28.071, -4.3254) (28.1967, -4.3568) (28.6521, -4.3568) knots 0 0 0 1 1 1
  line L21 (28.6521, -4.3568) -> (29.7829, -4.3568)
  line L22 (29.7829, -4.3568) -> (29.7829, -5.0573)
  line L23 (29.7829, -5.0573) -> (25.8755, -5.0573)
  line L24 (25.9729, -0.3112) -> (25.9729, 0.5494)
  spline S22 degree 2 poles (25.9729, 0.5494) (25.9729, 1.3817) (26.3843, 2.189) (27.3109, 2.7135) (27.9297, 2.7135) knots 0 0 0 1 2 3 3 3
  spline S23 degree 2 poles (27.9297, 2.7135) (28.3726, 2.7135) (29.1107, 2.4214) (29.5976, 1.9063) (29.7829, 1.3032) (29.7829, 0.5619) knots 0 0 0 1 2 3 4 4 4
  line L25 (29.7829, 0.5619) -> (29.7829, -0.3112)
  line L26 (29.7829, -0.3112) -> (25.9729, -0.3112)
  line L27 (26.6733, 0.408) -> (29.0762, 0.408)
  line L28 (29.0762, 0.408) -> (29.0762, 0.7473)
  spline S24 degree 2 poles (29.0762, 0.7473) (29.0762, 1.2467) (28.8469, 1.6958) (28.3098, 1.9817) (27.914, 1.9817) knots 0 0 0 1 2 3 3 3
  spline S25 degree 2 poles (27.914, 1.9817) (27.3078, 1.9817) (26.9748, 1.6424) knots 0 0 0 1 1 1
  spline S26 degree 2 poles (26.9748, 1.6424) (26.6733, 1.3346) (26.6733, 0.6562) knots 0 0 0 1 1 1
  line L29 (26.6733, 0.6562) -> (26.6733, 0.408)
  line L30 (28.5767, 6.1466) -> (28.5767, 3.8788)
  spline S27 degree 2 poles (28.5767, 3.8788) (28.8783, 3.9291) (29.2332, 4.3562) (29.2332, 4.686) knots 0 0 0 1 2 2 2
  spline S28 degree 2 poles (29.2332, 4.686) (29.2332, 5.0818) (28.9568, 5.3676) knots 0 0 0 1 1 1
  line L31 (28.9568, 5.3676) -> (29.2363, 5.9613)
  spline S29 degree 2 poles (29.2363, 5.9613) (29.5504, 5.7383) (29.8551, 5.1164) (29.8551, 4.6892) knots 0 0 0 1 2 2 2
  spline S30 degree 2 poles (29.8551, 4.6892) (29.8551, 4.0264) (29.0196, 3.1941) (28.3883, 3.1941) knots 0 0 0 1 2 2 2
  spline S31 degree 2 poles (28.3883, 3.1941) (27.7444, 3.1941) (26.8932, 4.0264) (26.8932, 4.6515) knots 0 0 0 1 2 2 2
  spline S32 degree 2 poles (26.8932, 4.6515) (26.8932, 5.3174) (27.7444, 6.1497) (28.4417, 6.1497) knots 0 0 0 1 2 2 2
  line L32 (28.4417, 6.1497) -> (28.5767, 6.1466)
  spline S33 degree 2 poles (28.0208, 5.4399) (27.7852, 5.3708) (27.4931, 4.9593) (27.4931, 4.686) knots 0 0 0 1 2 2 2
  spline S34 degree 2 poles (27.4931, 4.686) (27.4931, 4.3908) (27.6564, 4.1678) knots 0 0 0 1 1 1
  spline S35 degree 2 poles (27.6564, 4.1678) (27.7601, 4.0296) (28.0208, 3.9102) knots 0 0 0 1 1 1
  line L33 (28.0208, 3.9102) -> (28.0208, 5.4399)
  line L34 (27.5339, 9.4792) -> (27.8575, 8.8918)
  spline S36 degree 2 poles (27.8575, 8.8918) (27.6847, 8.7253) (27.5496, 8.4018) (27.5496, 8.1819) knots 0 0 0 1 2 2 2
  spline S37 degree 2 poles (27.5496, 8.1819) (27.5496, 7.7862) (28.0239, 7.2962) (28.3946, 7.2962) knots 0 0 0 1 2 2 2
  spline S38 degree 2 poles (28.3946, 7.2962) (28.7526, 7.2962) (29.2081, 7.7673) (29.2081, 8.1505) knots 0 0 0 1 2 2 2
  spline S39 degree 2 poles (29.2081, 8.1505) (29.2081, 8.6248) (28.8846, 8.8918) knots 0 0 0 1 1 1
  line L35 (28.8846, 8.8918) -> (29.2646, 9.4478)
  spline S40 degree 2 poles (29.2646, 9.4478) (29.8551, 8.9955) (29.8551, 8.1694) knots 0 0 0 1 1 1
  spline S41 degree 2 poles (29.8551, 8.1694) (29.8551, 7.425) (28.9756, 6.5832) (28.3851, 6.5832) knots 0 0 0 1 2 2 2
  spline S42 degree 2 poles (28.3851, 6.5832) (27.9768, 6.5832) (27.2858, 6.9915) (26.8932, 7.7265) (26.8932, 8.1788) knots 0 0 0 1 2 3 3 3
  spline S43 degree 2 poles (26.8932, 8.1788) (26.8932, 8.5997) (27.2261, 9.2656) (27.5339, 9.4792) knots 0 0 0 1 2 2 2
  line L36 (33.6771, -5.1295) -> (33.6771, -5.8362)
  spline S44 degree 2 poles (33.6771, -5.8362) (33.0615, -5.808) (32.3548, -5.0887) (32.3548, -4.5264) knots 0 0 0 1 2 2 2
  spline S45 degree 2 poles (32.3548, -4.5264) (32.3548, -4.1809) (32.6469, -3.647) (33.1997, -3.3297) (33.4824, -3.3297) knots 0 0 0 1 2 3 3 3
  spline S46 degree 2 poles (33.4824, -3.3297) (33.8216, -3.3297) (34.6037, -3.7161) (35.1377, -4.2312) knots 0 0 0 1 2 2 2
  line L37 (35.1377, -4.2312) -> (35.5868, -4.6584)
  line L38 (35.5868, -4.6584) -> (35.5868, -3.2983)
  line L39 (35.5868, -3.2983) -> (36.259, -3.2983)
  line L40 (36.259, -3.2983) -> (36.259, -5.9399)
  line L41 (36.259, -5.9399) -> (35.9135, -5.9399)
  line L42 (35.9135, -5.9399) -> (34.7105, -4.7589)
  spline S47 degree 2 poles (34.7105, -4.7589) (34.2771, -4.3317) (33.7525, -4.049) (33.5421, -4.049) knots 0 0 0 1 2 2 2
  spline S48 degree 2 poles (33.5421, -4.049) (33.3191, -4.049) (33.0332, -4.3411) (33.0332, -4.5735) knots 0 0 0 1 2 2 2
  spline S49 degree 2 poles (33.0332, -4.5735) (33.0332, -4.806) (33.3787, -5.1201) (33.6771, -5.1295) knots 0 0 0 1 2 2 2
  spline S50 degree 2 poles (32.3548, -1.6085) (32.3548, -1.1907) (32.7631, -0.5877) (33.6049, -0.2579) (34.3556, -0.2579) knots 0 0 0 1 2 3 3 3
  spline S51 degree 2 poles (34.3556, -0.2579) (35.1125, -0.2579) (35.9575, -0.5908) (36.3532, -1.1562) (36.3532, -1.5865) knots 0 0 0 1 2 3 3 3
  spline S52 degree 2 poles (36.3532, -1.5865) (36.3532, -2.0168) (35.9543, -2.601) (35.1408, -2.934) (34.3901, -2.934) knots 0 0 0 1 2 3 3 3
  spline S53 degree 2 poles (34.3901, -2.934) (33.3442, -2.934) (32.873, -2.6104) knots 0 0 0 1 1 1
  spline S54 degree 2 poles (32.873, -2.6104) (32.3548, -2.2492) (32.3548, -1.6085) knots 0 0 0 1 1 1
  spline S55 degree 2 poles (33.0426, -1.5896) (33.0426, -1.7749) (33.2782, -2.0576) (33.853, -2.2084) (34.4058, -2.2084) knots 0 0 0 1 2 3 3 3
  spline S56 degree 2 poles (34.4058, -2.2084) (35.1283, -2.2084) (35.6811, -1.866) (35.6811, -1.5896) knots 0 0 0 1 2 2 2
  spline S57 degree 2 poles (35.6811, -1.5896) (35.6811, -1.3258) (35.4204, -1.1719) knots 0 0 0 1 1 1
  spline S58 degree 2 poles (35.4204, -1.1719) (35.1031, -0.9834) (34.3619, -0.9834) knots 0 0 0 1 1 1
  spline S59 degree 2 poles (34.3619, -0.9834) (33.6112, -0.9834) (33.0426, -1.3226) (33.0426, -1.5896) knots 0 0 0 1 2 2 2
  line L43 (33.6771, 0.8132) -> (33.6771, 0.1065)
  spline S60 degree 2 poles (33.6771, 0.1065) (33.0615, 0.1348) (32.3548, 0.8541) (32.3548, 1.4163) knots 0 0 0 1 2 2 2
  spline S61 degree 2 poles (32.3548, 1.4163) (32.3548, 1.7618) (32.6469, 2.2958) (33.1997, 2.613) (33.4824, 2.613) knots 0 0 0 1 2 3 3 3
  spline S62 degree 2 poles (33.4824, 2.613) (33.8216, 2.613) (34.6037, 2.2267) (35.1377, 1.7115) knots 0 0 0 1 2 2 2
  line L44 (35.1377, 1.7115) -> (35.5868, 1.2844)
  line L45 (35.5868, 1.2844) -> (35.5868, 2.6444)
  line L46 (35.5868, 2.6444) -> (36.259, 2.6444)
  line L47 (36.259, 2.6444) -> (36.259, 0.0028)
  line L48 (36.259, 0.0028) -> (35.9135, 0.0028)
  line L49 (35.9135, 0.0028) -> (34.7105, 1.1839)
  spline S63 degree 2 poles (34.7105, 1.1839) (34.2771, 1.611) (33.7525, 1.8937) (33.5421, 1.8937) knots 0 0 0 1 2 2 2
  spline S64 degree 2 poles (33.5421, 1.8937) (33.3191, 1.8937) (33.0332, 1.6016) (33.0332, 1.3692) knots 0 0 0 1 2 2 2
  spline S65 degree 2 poles (33.0332, 1.3692) (33.0332, 1.1367) (33.3787, 0.8226) (33.6771, 0.8132) knots 0 0 0 1 2 2 2
  line L50 (32.449, 3.7469) -> (32.449, 5.531)
  line L51 (32.449, 5.531) -> (33.1212, 5.531)
  line L52 (33.1212, 5.531) -> (33.1212, 4.2871)
  line L53 (33.1212, 4.2871) -> (33.8122, 4.1332)
  spline S66 degree 2 poles (33.8122, 4.1332) (33.7933, 4.1992) (33.7745, 4.3217) (33.7745, 4.3782) knots 0 0 0 1 2 2 2
  spline S67 degree 2 poles (33.7745, 4.3782) (33.7745, 4.8965) (34.4812, 5.5844) (35.034, 5.5844) knots 0 0 0 1 2 2 2
  spline S68 degree 2 poles (35.034, 5.5844) (35.59, 5.5844) (36.3532, 4.8242) (36.3532, 4.2809) knots 0 0 0 1 2 2 2
  spline S69 degree 2 poles (36.3532, 4.2809) (36.3532, 3.794) (35.8004, 3.0967) (35.3199, 2.9868) knots 0 0 0 1 2 2 2
  line L54 (35.3199, 2.9868) -> (35.3199, 3.7469)
  spline S70 degree 2 poles (35.3199, 3.7469) (35.4989, 3.8348) (35.6811, 4.1238) (35.6811, 4.2966) knots 0 0 0 1 2 2 2
  spline S71 degree 2 poles (35.6811, 4.2966) (35.6811, 4.5384) (35.3356, 4.8745) (35.0623, 4.8745) knots 0 0 0 1 2 2 2
  spline S72 degree 2 poles (35.0623, 4.8745) (34.7985, 4.8745) (34.4592, 4.5604) (34.4592, 4.3374) knots 0 0 0 1 2 2 2
  spline S73 degree 2 poles (34.4592, 4.3374) (34.4592, 4.218) (34.5786, 3.9887) (34.6979, 3.8788) knots 0 0 0 1 2 2 2
  line L55 (34.6979, 3.8788) -> (34.566, 3.2852)
  line L56 (34.566, 3.2852) -> (32.449, 3.7469)
  point P0 (0, 0)
  dimension "d0" = 40
  dimension "d30" = 102
  constraints: 2 other
emboss "Emboss1" sketch "Sketch6" operation cut depth 1.5 direction (1, 0, 0)
emboss "Emboss2" [suppressed]
emboss "Emboss3" sketch "Sketch8" operation cut depth 1.5 direction (1, 0, 0)
fillet "Fillet1" radius 1 16 edges at (88.5, 0, 51) (0, 0, 51) (88.5, 0, -51) (0, 0, -51) (44.25, 20, -51) (88.5, 20, -27.125) (88.5, 20, 27.125) (44.25, 20, 51) (0, 20, 27.125) (0, 20, -27.125) (0, -20, -27.125) (0, -20, 27.125) (44.25, -20, 51) (88.5, -20, 27.125) (88.5, -20, -27.125) (44.25, -20, -51)
fillet "Fillet2" radius 2 8 edges at (3.2209, -11, -3.25) (3.2209, -11, 3.25) (85.7209, -11, -3.25) (85.7209, -11, 3.25) (85.7209, 11, 3.25) (85.7209, 11, -3.25) (3.2209, 11, 3.25) (3.2209, 11, -3.25)
body "Solid1"
